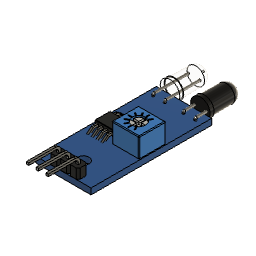
HW-201 v4 (Autodesk Fusion 360 design; units mm, degrees)
Autodesk Fusion 360 part; units mm, degrees
note: some values were not read from the file. Chosen so that the rebuilt part matches the saved one: which bodies a step acts on. Set by a fixed rule: which sketch regions a step uses.
sketch "Sketch1" plane through (0, 0, 0) normal (0, 0, 1) x (1, 0, 0)
  line L0 (7.1, 15.5) -> (-7.1, 15.5)
  line L1 (-7.1, 15.5) -> (-7.1, -15.5)
  line L2 (-7.1, -15.5) -> (7.1, -15.5)
  line L3 (7.1, -15.5) -> (7.1, 15.5)
  line L4 (7.1, 15.5) -> (-7.1, -15.5) construction
  line L5 (-7.1, 15.5) -> (7.1, -15.5) construction
  circle A0 centre (0, -10.4) radius 1.5
  line L6 (0, -10.4) -> (0, -15.5) construction
  dimension "d1" = 14.2
  dimension "d2" = 31
  dimension "d3" = 3
  dimension "d4" = 5.1
  constraint horizontal L0
  constraint perpendicular L0 L1
  constraint parallel L0 L2
  constraint parallel L1 L3
  constraint coincident L4 origin
  constraint coincident L5 origin
  constraint coincident A0.centre L6.start
  constraint midpoint L2 L6.end
  constraint vertical L6
  measures "d1" distance of L1.end L2.end
  measures "d2" distance of L0.end L1.end
  measures "d3" diameter of A0
  measures "d4" distance of A0.centre L6.end
extrude "Extrude1" add sketch "Sketch1" along normal blind 1.54 contours L0 L1 L2 L3 picked at (0.037365, 7.365269) makes body 1
sketch "Sketch2" plane through (0, 0, 1.54) normal (0, 0, 1) x (-1, 0, 0)
  circle A0 centre (0, 10.4) radius 1.5
  line L0 (-7.1, 15.5) -> (-7.1, -15.5)
  line L1 (-7.1, -15.5) -> (7.1, -15.5)
  line L2 (7.1, -15.5) -> (7.1, 15.5)
  line L3 (7.1, 15.5) -> (-7.1, 15.5)
  line L4 (-1.75, 12.95) -> (-3.25, 12.95)
  line L5 (-3.25, 12.95) -> (-3.25, 15.45) construction
  line L6 (-3.25, 15.45) -> (-1.75, 15.45)
  line L7 (-1.75, 15.45) -> (-1.75, 12.95) construction
  line L8 (-1.25, 13.45) -> (-3.75, 13.45) construction
  line L9 (-3.75, 13.45) -> (-3.75, 14.95)
  line L10 (-3.75, 14.95) -> (-1.25, 14.95) construction
  line L11 (-1.25, 14.95) -> (-1.25, 13.45)
  line L12 (1.25, 13.45) -> (-1.25, 13.45) construction
  line L13 (-1.25, 13.45) -> (-1.25, 14.95)
  line L14 (-1.25, 14.95) -> (1.25, 14.95) construction
  line L15 (1.25, 14.95) -> (1.25, 13.45)
  line L16 (0.75, 12.95) -> (-0.75, 12.95)
  line L17 (-0.75, 12.95) -> (-0.75, 15.45) construction
  line L18 (-0.75, 15.45) -> (0.75, 15.45)
  line L19 (0.75, 15.45) -> (0.75, 12.95) construction
  line L20 (3.75, 13.45) -> (1.25, 13.45) construction
  line L21 (1.25, 13.45) -> (1.25, 14.95)
  line L22 (1.25, 14.95) -> (3.75, 14.95) construction
  line L23 (3.75, 14.95) -> (3.75, 13.45)
  line L24 (3.25, 12.95) -> (1.75, 12.95)
  line L25 (1.75, 12.95) -> (1.75, 15.45) construction
  line L26 (1.75, 15.45) -> (3.25, 15.45)
  line L27 (3.25, 15.45) -> (3.25, 12.95) construction
  line L28 (0.75, 12.95) -> (1.25, 13.45)
  line L29 (1.75, 12.95) -> (1.25, 13.45)
  line L30 (3.25, 12.95) -> (3.75, 13.45)
  line L31 (3.75, 14.95) -> (3.25, 15.45)
  line L32 (1.75, 15.45) -> (1.25, 14.95)
  line L33 (1.25, 14.2) -> (3.75, 14.2) construction
  line L34 (2.5, 12.95) -> (2.5, 15.45) construction
  line L35 (0, 12.95) -> (0, 15.45) construction
  line L36 (1.25, 14.2) -> (-1.25, 14.2) construction
  line L37 (-0.75, 12.95) -> (-1.25, 13.45)
  line L38 (-1.25, 14.95) -> (-0.75, 15.45)
  line L39 (1.25, 14.95) -> (0.75, 15.45)
  line L40 (-1.25, 13.45) -> (-1.75, 12.95)
  line L41 (-3.25, 12.95) -> (-3.75, 13.45)
  line L42 (-3.75, 14.95) -> (-3.25, 15.45)
  line L43 (-1.75, 15.45) -> (-1.25, 14.95)
  line L44 (-2.5, 12.95) -> (-2.5, 15.45) construction
  line L45 (-1.25, 14.2) -> (-3.75, 14.2) construction
  line L46 (0, 15.5) -> (0, 14.2) construction
  dimension "d7" = 45
  dimension "d8" = 2.5
  dimension "d9" = 2.5
  dimension "d10" = 2.5
  dimension "d11" = 2.5
  dimension "d12" = 2.5
  dimension "d13" = 2.5
  dimension "d14" = 45
  dimension "d15" = 45
  dimension "d16" = 0.5
  dimension "d17" = 0.5
  dimension "d18" = 0.5
  dimension "d20" = 0.05
  constraint horizontal L4
  constraint vertical L5
  constraint horizontal L6
  constraint vertical L7
  constraint horizontal L8
  constraint vertical L9
  constraint horizontal L10
  constraint vertical L11
  constraint horizontal L12
  constraint vertical L13
  constraint horizontal L14
  constraint vertical L15
  constraint horizontal L16
  constraint vertical L17
  constraint horizontal L18
  constraint vertical L19
  constraint horizontal L20
  constraint vertical L21
  constraint horizontal L22
  constraint vertical L23
  constraint horizontal L24
  constraint vertical L25
  constraint horizontal L26
  constraint vertical L27
  constraint midpoint L21 L33.start
  constraint midpoint L23 L33.end
  constraint midpoint L24 L34.start
  constraint midpoint L26 L34.end
  constraint midpoint L16 L35.start
  constraint perpendicular L16 L35
  constraint midpoint L15 L33.start
  constraint midpoint L13 L36.end
  constraint perpendicular L13 L36
  constraint midpoint L4 L44.start
  constraint midpoint L6 L44.end
  constraint midpoint L11 L36.end
  constraint midpoint L9 L45.end
  constraint midpoint L35 L36
  constraint midpoint L44 L45
  constraint midpoint L33 L34
  constraint coincident L18 L35.end
  constraint collinear L11 L13
  constraint collinear L15 L21
  constraint collinear L4 L16
  constraint collinear L16 L24
  constraint midpoint L3 L46.start
  constraint midpoint L35 L46.end
  constraint vertical L46
  measures "d7" angle of L19 L28
  measures "d8" distance of L8.start L8.end
  measures "d9" distance of L44.start L44.end
  measures "d10" distance of L16.end L17.end
  measures "d11" distance of L12.start L8.start
  measures "d12" distance of L20.start L12.start
  measures "d13" distance of L24.end L25.end
  measures "d14" angle of L7 L40
  measures "d15" angle of L27 L30
  measures "d16" distance of L15 L19
  measures "d17" distance of L7 L11
  measures "d18" distance of L21 L25
  measures "d20" distance of L3 L18
sketch "Sketch3" plane through (0, 0, 1.54) normal (0, 0, 1) x (1, 0, 0)
  line L0 (-0.15, 3.95) -> (6.85, 3.95)
  line L1 (6.85, 3.95) -> (6.85, -2.9)
  line L2 (6.85, -2.9) -> (-0.15, -2.9)
  line L3 (-0.15, -2.9) -> (-0.15, 3.95)
  line L4 (-7.1, -15.5) -> (7.1, -15.5)
  line L5 (7.1, -15.5) -> (7.1, 15.5)
  dimension "d21" = 6.85
  dimension "d22" = 7
  dimension "d23" = 19.45
  dimension "d24" = 0.25
  constraint horizontal L0
  constraint vertical L1
  constraint horizontal L2
  constraint vertical L3
  measures "d21" distance of L0.end L1.end
  measures "d22" distance of L0.start L0.end
  measures "d23" distance of L0 L4
  measures "d24" distance of L1 L5
extrude "Extrude2" add sketch "Sketch3" along normal blind 5 separate body contours L0 L1 L2 L3 picked at (2.183333, 1.666667) makes body 2
sketch "Sketch4" plane through (0, 0, 6.54) normal (0, 0, 1) x (-1, 0, 0)
  line L0 (0.15, 2.9) -> (-6.85, 2.9)
  line L1 (-6.85, 2.9) -> (-6.85, -3.95)
  line L2 (-6.85, -3.95) -> (0.15, -3.95)
  line L3 (0.15, -3.95) -> (0.15, 2.9)
  line L4 (0.15, -0.525) -> (-6.85, -0.525) construction
  line L5 (-3.35, -3.95) -> (-3.35, 2.9) construction
  circle A0 centre (-3.35, -0.525) radius 1.75
  line L6 (-3.25, -3.272141) -> (-3.45, -3.272141)
  line L7 (-3.45, -3.272141) -> (-3.45, -2.272141)
  line L8 (-3.45, -2.272141) -> (-3.25, -2.272141)
  line L9 (-3.25, -2.272141) -> (-3.25, -3.272141)
  line L10 (-3.35, -3.272141) -> (-3.35, -2.272141) construction
  line L11 (-2.063032, -2.954093) -> (-2.563032, -2.088068)
  line L12 (-2.389827, -1.988068) -> (-1.889827, -2.854093)
  line L13 (-1.889827, -2.854093) -> (-2.063032, -2.954093)
  line L14 (-1.020907, -1.985173) -> (-1.886932, -1.485173)
  line L15 (-1.786932, -1.311968) -> (-0.920907, -1.811968)
  line L16 (-0.920907, -1.811968) -> (-1.020907, -1.985173)
  line L17 (-0.602859, -0.625) -> (-1.602859, -0.625)
  line L18 (-1.602859, -0.425) -> (-0.602859, -0.425)
  line L19 (-0.602859, -0.425) -> (-0.602859, -0.625)
  line L20 (-0.920907, 0.761968) -> (-1.786932, 0.261968)
  line L21 (-1.886932, 0.435173) -> (-1.020907, 0.935173)
  line L22 (-1.020907, 0.935173) -> (-0.920907, 0.761968)
  line L23 (-4.810173, -2.854093) -> (-4.310173, -1.988068)
  line L24 (-4.136968, -2.088068) -> (-4.636968, -2.954093)
  line L25 (-4.636968, -2.954093) -> (-4.810173, -2.854093)
  line L26 (-1.889827, 1.804093) -> (-2.389827, 0.938068)
  line L27 (-2.563032, 1.038068) -> (-2.063032, 1.904093)
  line L28 (-2.063032, 1.904093) -> (-1.889827, 1.804093)
  line L29 (-3.25, 2.222141) -> (-3.25, 1.222141)
  line L30 (-3.45, 1.222141) -> (-3.45, 2.222141)
  line L31 (-3.45, 2.222141) -> (-3.25, 2.222141)
  line L32 (-4.636968, 1.904093) -> (-4.136968, 1.038068)
  line L33 (-4.310173, 0.938068) -> (-4.810173, 1.804093)
  line L34 (-4.810173, 1.804093) -> (-4.636968, 1.904093)
  dimension "d27" = 3.5
  dimension "d28" = 0.2
  dimension "d29" = 1
  dimension "d31" = 360
  constraint midpoint L3 L4.start
  constraint midpoint L1 L4.end
  constraint midpoint L2 L5.start
  constraint midpoint L0 L5.end
  constraint midpoint L4 A0.centre
  constraint horizontal L6
  constraint vertical L7
  constraint horizontal L8
  constraint vertical L9
  constraint perpendicular L8 L10
  measures "d27" diameter of A0
extrude "Extrude3" cut sketch "Sketch4" against normal blind 2 contours A0 L8 picked at (-2.629228, -0.607791) bodies 2
extrude "Extrude4" cut sketch "Sketch4" against normal blind 0.1 contours A0 L17 L18 L19 | A0 L20 L21 L22 | A0 L14 L15 L16 | A0 L26 L27 L28 | A0 L11 L12 L13 | A0 L29 L30 L31 | A0 L6 L7 L9 | A0 L32 L33 L34 | A0 L23 L24 L25 picked at (-0.93524, -0.525) picked at (-1.25329, 0.6727) picked at (-1.264406, -1.741954) picked at (-2.1523, 1.57171) picked at (-2.133046, -2.610594) picked at (-3.361116, 1.889654) picked at (-3.338884, -2.939654) picked at (-4.5477, 1.57171) picked at (-4.5477, -2.62171) bodies 2
sketch "Sketch5" plane through (0, 0, 4.54) normal (0, 0, 1) x (-1, 0, 0)
  line L0 (-3.45, -2.272141) -> (-3.25, -2.272141)
  arc A0 (-3.25, -2.272141) -> (-3.45, -2.272141) centre (-3.35, -0.525) ccw
  circle A1 centre (-3.35, -0.525) radius 1.747141
  constraint concentric A0 A1
  constraint tangent L0 A1
extrude "Extrude5" add sketch "Sketch5" along normal blind 1.6 separate body contours L0 A0 A1 picked at (-3.907573, -0.499504) makes body 3
sketch "Sketch6" plane through (0, 0, 6.14) normal (0, 0, 1) x (-1, 0, 0)
  circle A0 centre (-3.35, -0.525) radius 1.747141
  line L0 (-5.097141, -0.8698) -> (-5.097141, -0.1802)
  line L1 (-1.602859, -0.1802) -> (-1.602859, -0.8698)
  line L2 (-3.01881, -2.272141) -> (-3.68119, -2.272141)
  line L3 (-3.68119, 1.222141) -> (-3.01881, 1.222141)
  circle A1 centre (-3.35, -0.525) radius 1.747141
  line L4 (-3.35, -0.525) -> (-3.35, -2.272141) construction
  line L5 (-3.35, -0.525) -> (-1.602859, -0.525) construction
  line L6 (-3.01881, -2.272141) -> (-3.01881, -0.8698)
  line L7 (-3.01881, -0.1802) -> (-3.01881, 1.222141)
  line L8 (-3.68119, 1.222141) -> (-3.68119, -0.1802)
  line L9 (-3.68119, -0.8698) -> (-3.68119, -2.272141)
  line L10 (-1.602859, -0.8698) -> (-3.01881, -0.8698)
  line L11 (-3.68119, -0.8698) -> (-5.097141, -0.8698)
  line L12 (-5.097141, -0.1802) -> (-3.68119, -0.1802)
  line L13 (-3.01881, -0.1802) -> (-1.602859, -0.1802)
  constraint vertical L8
  constraint horizontal L10
  constraint perpendicular L0 L10
  constraint perpendicular L0 L12
  constraint vertical L6
  constraint horizontal L2
  constraint vertical L1
  constraint horizontal L3
  constraint concentric A0 A1
  constraint coincident A0.centre A1.centre
  constraint vertical L4
  constraint horizontal L5
  constraint tangent L2 A1
  constraint tangent L1 A1
  constraint tangent L3 A1
  constraint tangent L0 A1
  constraint collinear L6 L7
  constraint collinear L8 L9
  constraint collinear L10 L11
  constraint collinear L12 L13
extrude "Extrude6" cut sketch "Sketch6" against normal blind 0.5 contours A0 A1 L6 L7 L8 L9 L10 L11 L12 L13 picked at (-2.546827, -0.525) bodies 3
extrude "Extrude7" add sketch "Sketch2" along normal blind 2.5 separate body contours L4 L6 L9 L11 L13 L40 L41 L42 L43 | L11 L13 L15 L16 L18 L21 L28 L37 L38 L39 | L15 L21 L23 L24 L26 L29 L30 L31 L32 picked at (-2.75, 14.616667) picked at (-0.083333, 13.95) picked at (2.75, 13.783333) makes body 4
sketch "Sketch7" plane through (0, 0, 4.04) normal (0, 0, 1) x (-1, 0, 0)
  line L0 (0.75, 12.95) -> (1.25, 13.45)
  line L1 (1.25, 13.45) -> (1.75, 12.95)
  line L2 (1.75, 12.95) -> (3.25, 12.95)
  line L3 (3.25, 12.95) -> (3.75, 13.45)
  line L4 (3.75, 13.45) -> (3.75, 14.95)
  line L5 (3.75, 14.95) -> (3.25, 15.45)
  line L6 (3.25, 15.45) -> (1.75, 15.45)
  line L7 (1.75, 15.45) -> (1.25, 14.95)
  line L8 (1.25, 14.95) -> (0.75, 15.45)
  line L9 (0.75, 15.45) -> (-0.75, 15.45)
  line L10 (-0.75, 15.45) -> (-1.25, 14.95)
  line L11 (-1.25, 14.95) -> (-1.75, 15.45)
  line L12 (-1.75, 15.45) -> (-3.25, 15.45)
  line L13 (-3.25, 15.45) -> (-3.75, 14.95)
  line L14 (-3.75, 14.95) -> (-3.75, 13.45)
  line L15 (-3.75, 13.45) -> (-3.25, 12.95)
  line L16 (-3.25, 12.95) -> (-1.75, 12.95)
  line L17 (-1.75, 12.95) -> (-1.25, 13.45)
  line L18 (-1.25, 13.45) -> (-0.75, 12.95)
  line L19 (-0.75, 12.95) -> (0.75, 12.95)
  line L20 (2.8, 13.9) -> (2.2, 13.9)
  line L21 (2.2, 13.9) -> (2.2, 14.5)
  line L22 (2.2, 14.5) -> (2.8, 14.5)
  line L23 (2.8, 14.5) -> (2.8, 13.9)
  line L24 (0.3, 13.9) -> (-0.3, 13.9)
  line L25 (-0.3, 13.9) -> (-0.3, 14.5)
  line L26 (-0.3, 14.5) -> (0.3, 14.5)
  line L27 (0.3, 14.5) -> (0.3, 13.9)
  line L28 (-2.2, 13.9) -> (-2.8, 13.9)
  line L29 (-2.8, 13.9) -> (-2.8, 14.5)
  line L30 (-2.8, 14.5) -> (-2.2, 14.5)
  line L31 (-2.2, 14.5) -> (-2.2, 13.9)
  line L32 (2.5, 12.95) -> (2.5, 15.45) construction
  line L33 (3.75, 14.2) -> (-3.75, 14.2) construction
  line L34 (-2.5, 12.95) -> (-2.5, 15.45) construction
  line L35 (0, 12.95) -> (0, 15.45) construction
  line L36 (-2.5, 13.9) -> (-2.5, 14.5) construction
  line L37 (0.3, 14.2) -> (-0.3, 14.2) construction
  line L38 (2.5, 14.5) -> (2.5, 13.9) construction
  line L39 (0, 14.5) -> (0, 13.9) construction
  dimension "d42" = 0.6
  constraint horizontal L20
  constraint vertical L21
  constraint horizontal L22
  constraint vertical L23
  constraint horizontal L24
  constraint vertical L25
  constraint horizontal L26
  constraint vertical L27
  constraint horizontal L28
  constraint vertical L29
  constraint horizontal L30
  constraint vertical L31
  constraint equal L28 L29
  constraint equal L24 L25
  constraint equal L20 L21
  constraint equal L20 L24
  constraint equal L24 L28
  constraint midpoint L2 L32.start
  constraint midpoint L6 L32.end
  constraint midpoint L4 L33.start
  constraint midpoint L14 L33.end
  constraint midpoint L16 L34.start
  constraint midpoint L12 L34.end
  constraint midpoint L19 L35.start
  constraint midpoint L9 L35.end
  constraint midpoint L28 L36.start
  constraint midpoint L30 L36.end
  constraint perpendicular L30 L36
  constraint midpoint L27 L37.start
  constraint midpoint L25 L37.end
  constraint midpoint L22 L38.start
  constraint midpoint L20 L38.end
  constraint perpendicular L20 L38
  constraint collinear L24 L28
  constraint collinear L20 L24
  constraint collinear L34 L36
  constraint midpoint L26 L39.start
  constraint midpoint L24 L39.end
  constraint collinear L35 L39
  constraint collinear L32 L38
  constraint collinear L33 L37
  measures "d42" distance of L28.start L28.end
sketch "Sketch8" plane through (3.75, 0, 0) normal (1, 0, 0) x (0, 1, 0)
  line L0 (-14.95, 1.54) -> (-13.45, 1.54)
  line L1 (-13.45, 1.54) -> (-13.45, 4.04)
  line L2 (-13.45, 4.04) -> (-14.95, 4.04)
  line L3 (-14.95, 4.04) -> (-14.95, 1.54)
  line L4 (-14.2, 4.04) -> (-14.2, 4.54)
  line L5 (-15.2, 5.54) -> (-22.2, 5.54)
  arc A0 (-14.2, 4.54) -> (-15.2, 5.54) centre (-15.2, 4.54) ccw
  point P0 (-14.2, 5.54)
  dimension "d43" = 1.5
  dimension "d44" = 8
  dimension "d45" = 1
  constraint midpoint L2 L4.start
  constraint perpendicular L2 L4
  constraint perpendicular L4 L5
  constraint coincident P0 L5
  constraint coincident P0 L4
  constraint tangent L5 A0
  constraint tangent L4 A0
  measures "d43" distance of L4.start P0
  measures "d44" distance of P0 L5.end
  measures "d45" radius of A0
sweep "Sweep1" add profiles "Sketch7" path "Sketch8" along L4 A0 L5 section 1 contours L20 L21 L22 L23 | L24 L25 L26 L27 | L28 L29 L30 L31 picked at (2.6, 14.1) picked at (0.1, 14.1) picked at (-2.4, 14.1) separate body makes body 5 at (2.8, -17.533333, 5.44) makes body 6 at (0.3, -17.533333, 5.44) makes body 7 at (-2.2, -17.533333, 5.44)
sketch "Sketch9" plane through (7.1, 0, 0) normal (1, 0, 0) x (0, 1, 0)
  line L0 (-15.5, 0) -> (15.5, 0)
  line L1 (15.5, 0) -> (15.5, 1.54)
  line L2 (15.5, 1.54) -> (-15.5, 1.54)
  line L3 (-15.5, 1.54) -> (-15.5, 0)
  line L4 (13, -2.3) -> (13, 2.04) construction
  line L5 (13.2, 2.04) -> (22, 2.04)
  line L6 (13, 1.84) -> (13, 1.54)
  line L7 (13, 0) -> (13, -2.3)
  arc A0 (13.2, 2.04) -> (13, 1.84) centre (13.2, 1.84) ccw
  dimension "d52" = 2.5
  dimension "d53" = 0.5
  dimension "d54" = 2.3
  dimension "d55" = 9
  dimension "d69" = 0.2
  constraint perpendicular L0 L4
  constraint perpendicular L4 L5
  constraint coincident L4 L6.end
  constraint coincident L2 L6.end
  constraint coincident L0 L7.start
  constraint coincident L4 L7.start
  constraint coincident L4.end L6
  constraint coincident L4.end L5
  constraint tangent L5 A0
  measures "d52" distance of L1 L4
  measures "d53" distance of L2 L5
  measures "d54" distance of L0 L4.start
  measures "d55" distance of L4.end L5.end
  measures "d69" radius of A0
sketch "Sketch10" plane through (0, 0, 1.54) normal (0, 0, 1) x (-1, 0, 0)
  circle A0 centre (0, 10.4) radius 1.5
  line L0 (-7.1, 15.5) -> (-7.1, -15.5)
  line L1 (-7.1, -15.5) -> (7.1, -15.5)
  line L2 (7.1, -15.5) -> (7.1, 15.5)
  line L3 (7.1, 15.5) -> (-7.1, 15.5)
  line L4 (-3.9, -14.5) -> (-6.9, -14.5)
  line L5 (-6.9, -14.5) -> (-6.9, -11.5)
  line L6 (-6.9, -11.5) -> (-3.9, -11.5)
  line L7 (-3.9, -11.5) -> (-3.9, -14.5)
  line L8 (-0.9, -14.5) -> (-3.9, -14.5)
  line L9 (-3.9, -14.5) -> (-3.9, -11.5)
  line L10 (-3.9, -11.5) -> (-0.9, -11.5)
  line L11 (-0.9, -11.5) -> (-0.9, -14.5)
  line L12 (3.9, -14.5) -> (0.9, -14.5)
  line L13 (0.9, -14.5) -> (0.9, -11.5)
  line L14 (0.9, -11.5) -> (3.9, -11.5)
  line L15 (3.9, -11.5) -> (3.9, -14.5)
  line L16 (6.9, -14.5) -> (3.9, -14.5)
  line L17 (3.9, -14.5) -> (3.9, -11.5)
  line L18 (3.9, -11.5) -> (6.9, -11.5)
  line L19 (6.9, -11.5) -> (6.9, -14.5)
  line L20 (-7.1, -13) -> (7.1, -13) construction
  line L21 (-7.1, -13.2) -> (-7.1, -22)
  line L22 (-5.1, -13.3) -> (-5.7, -13.3) construction
  line L23 (-5.7, -13.3) -> (-5.7, -12.7) construction
  line L24 (-5.7, -12.7) -> (-5.1, -12.7) construction
  line L25 (-5.1, -12.7) -> (-5.1, -13.3) construction
  line L26 (-2.1, -13.3) -> (-2.7, -13.3) construction
  line L27 (-2.7, -13.3) -> (-2.7, -12.7) construction
  line L28 (-2.7, -12.7) -> (-2.1, -12.7) construction
  line L29 (-2.1, -12.7) -> (-2.1, -13.3) construction
  line L30 (2.7, -13.3) -> (2.1, -13.3) construction
  line L31 (2.1, -13.3) -> (2.1, -12.7) construction
  line L32 (2.1, -12.7) -> (2.7, -12.7) construction
  line L33 (2.7, -12.7) -> (2.7, -13.3) construction
  line L34 (5.7, -13.3) -> (5.1, -13.3) construction
  line L35 (5.1, -13.3) -> (5.1, -12.7) construction
  line L36 (5.1, -12.7) -> (5.7, -12.7) construction
  line L37 (5.7, -12.7) -> (5.7, -13.3) construction
  line L38 (-2.4, -14.5) -> (-2.4, -11.5) construction
  line L39 (-5.4, -14.5) -> (-5.4, -11.5) construction
  line L40 (2.4, -14.5) -> (2.4, -11.5) construction
  line L41 (5.4, -14.5) -> (5.4, -11.5) construction
  line L42 (5.7, -13) -> (5.1, -13) construction
  line L43 (5.4, -13.3) -> (5.4, -12.7) construction
  line L44 (2.4, -13.3) -> (2.4, -12.7) construction
  line L45 (2.7, -13) -> (2.1, -13) construction
  line L46 (-2.4, -13.3) -> (-2.4, -12.7) construction
  line L47 (-5.4, -13.3) -> (-5.4, -12.7) construction
  circle A1 centre (5.4, -13) radius 0.3
  circle A2 centre (2.4, -13) radius 0.3
  circle A3 centre (-2.4, -13) radius 0.3
  circle A4 centre (-5.4, -13) radius 0.3
  line L48 (4, -11.6) -> (6.8, -11.6)
  line L49 (6.8, -11.6) -> (6.8, -14.4)
  line L50 (6.8, -14.4) -> (4, -14.4)
  line L51 (4, -14.4) -> (4, -11.6)
  line L52 (1, -11.6) -> (3.8, -11.6)
  line L53 (3.8, -11.6) -> (3.8, -14.4)
  line L54 (3.8, -14.4) -> (1, -14.4)
  line L55 (1, -14.4) -> (1, -11.6)
  line L56 (-3.8, -11.6) -> (-1, -11.6)
  line L57 (-1, -11.6) -> (-1, -14.4)
  line L58 (-1, -14.4) -> (-3.8, -14.4)
  line L59 (-3.8, -14.4) -> (-3.8, -11.6)
  line L60 (-6.8, -11.6) -> (-4, -11.6)
  line L61 (-4, -11.6) -> (-4, -14.4)
  line L62 (-4, -14.4) -> (-6.8, -14.4)
  line L63 (-6.8, -14.4) -> (-6.8, -11.6)
  point P0 (-7.1, -13)
  dimension "d56" = 3
  dimension "d57" = 3
  dimension "d58" = 3
  dimension "d59" = 1
  dimension "d60" = 0.2
  dimension "d61" = 3
  dimension "d62" = 3
  dimension "d63" = 0.2
  dimension "d64" = 0.6
  dimension "d65" = 0.1
  dimension "d66" = 0.1
  dimension "d67" = 0.1
  dimension "d68" = 0.1
  constraint horizontal L4
  constraint vertical L5
  constraint horizontal L6
  constraint vertical L7
  constraint horizontal L8
  constraint vertical L9
  constraint horizontal L10
  constraint vertical L11
  constraint horizontal L12
  constraint vertical L13
  constraint horizontal L14
  constraint vertical L15
  constraint horizontal L16
  constraint vertical L17
  constraint horizontal L18
  constraint vertical L19
  constraint collinear L15 L17
  constraint collinear L14 L18
  constraint collinear L12 L16
  constraint perpendicular L2 L20
  constraint collinear L8 L12
  constraint collinear L4 L12
  constraint collinear L10 L14
  constraint collinear L6 L10
  constraint collinear L7 L9
  constraint horizontal L22
  constraint vertical L23
  constraint horizontal L24
  constraint vertical L25
  constraint horizontal L26
  constraint vertical L27
  constraint horizontal L28
  constraint vertical L29
  constraint horizontal L30
  constraint vertical L31
  constraint horizontal L32
  constraint vertical L33
  constraint horizontal L34
  constraint vertical L35
  constraint horizontal L36
  constraint vertical L37
  constraint equal L34 L35
  constraint equal L30 L34
  constraint equal L30 L31
  constraint equal L26 L30
  constraint equal L26 L27
  constraint equal L25 L27
  constraint equal L22 L25
  constraint collinear L30 L34
  constraint collinear L26 L30
  constraint collinear L22 L26
  constraint midpoint L8 L38.start
  constraint midpoint L10 L38.end
  constraint midpoint L4 L39.start
  constraint midpoint L6 L39.end
  constraint midpoint L12 L40.start
  constraint midpoint L14 L40.end
  constraint midpoint L16 L41.start
  constraint midpoint L18 L41.end
  constraint midpoint L37 L42.start
  constraint midpoint L35 L42.end
  constraint midpoint L34 L43.start
  constraint midpoint L36 L43.end
  constraint perpendicular L36 L43
  constraint midpoint L30 L44.start
  constraint midpoint L32 L44.end
  constraint midpoint L33 L45.start
  constraint midpoint L31 L45.end
  constraint collinear L20 L42
  constraint midpoint L26 L46.start
  constraint midpoint L28 L46.end
  constraint collinear L38 L46
  constraint midpoint L22 L47.start
  constraint midpoint L24 L47.end
  constraint perpendicular L24 L47
  constraint collinear L39 L47
  constraint collinear L40 L44
  constraint collinear L41 L43
  constraint midpoint L42 A1.centre
  constraint coincident L43.start A1
  constraint midpoint L40 A2.centre
  constraint coincident L44.start A2
  constraint midpoint L38 A3.centre
  constraint coincident L46.start A3
  constraint midpoint L47 A4.centre
  constraint coincident L47.start A4
  constraint coincident L2 L20.end
  constraint coincident P0 L20.start
  measures "d56" distance of L16.start L12.start
  measures "d57" distance of L12.start L12.end
  measures "d58" distance of L16.start L18.end
  measures "d59" distance of L1 L16
  measures "d60" distance of L2 L19
  measures "d61" distance of L4.start L4.end
  measures "d62" distance of L8.start L4.start
  measures "d63" distance of L5 L21
  measures "d64" distance of L32.end L31
sweep "Sweep2" add profiles "Sketch10" path "Sketch9" along L5 A0 L6 section 1 contours A1 | A2 | A3 | A4 picked at (5.272872, -13.056332) picked at (2.488251, -12.931983) picked at (-2.311749, -12.931983) picked at (-5.527128, -13.056332) separate body makes body 8 at (5.630983, 19.066667, 1.848567) makes body 9 at (2.630983, 19.066667, 1.848567) makes body 10 at (-5.169017, 19.066667, 1.848567) makes body 11 at (-2.169017, 19.066667, 1.848567)
ref_plane "WorkPlane1" through (0, 15.8, 0.77) normal (0, 1, 0) x (-1, 0, 0)
sketch "Sketch11" plane through (0, 15.8, 0.77) normal (0, 1, 0) x (1, 0, 0)
  circle A0 centre (5.4, -1.27) radius 0.3
  circle A1 centre (2.4, -1.27) radius 0.3
  line L0 (7.1, 0.77) -> (-7.1, 0.77)
  line L1 (-7.1, 0.77) -> (-7.1, -0.77)
  line L2 (-7.1, -0.77) -> (7.1, -0.77)
  line L3 (7.1, -0.77) -> (7.1, 0.77)
  line L4 (5.4, -1.27) -> (2.4, -1.27) construction
  line L5 (3.9, -3.77) -> (3.9, 1.23) construction
  circle A2 centre (3.9, -1.27) radius 2.5
  circle A3 centre (-2.4, -1.27) radius 0.3
  circle A4 centre (-5.4, -1.27) radius 0.3
  line L6 (-7.1, 0.77) -> (7.1, 0.77)
  line L7 (7.1, 0.77) -> (7.1, -0.77)
  line L8 (7.1, -0.77) -> (-7.1, -0.77)
  line L9 (-7.1, -0.77) -> (-7.1, 0.77)
  line L10 (-2.4, -1.27) -> (-5.4, -1.27) construction
  line L11 (-3.9, -3.77) -> (-3.9, 1.23) construction
  circle A5 centre (-3.9, -1.27) radius 2.5
  dimension "d77" = 5
  dimension "d78" = 5
  constraint coincident A0.centre L4.start
  constraint coincident A1.centre L4.end
  constraint perpendicular L2 L5
  constraint midpoint L4 L5
  constraint midpoint L4 A2.centre
  constraint coincident L5.start A2
  constraint coincident A3.centre L10.start
  constraint coincident A4.centre L10.end
  constraint perpendicular L0 L11
  constraint midpoint L10 L11
  constraint midpoint L10 A5.centre
  constraint coincident L11.start A5
  measures "d77" distance of L5.start L5.end
  measures "d78" distance of L11.start L11.end
extrude "Extrude8" add sketch "Sketch11" along normal blind 1 separate body contours A0 | A1 | L0 L2 A2 L6 L8 | L0 A2 L6 | L2 A2 L8 | L0 L2 L6 L8 A5 | L0 L6 A5 | L2 L8 A5 | A3 | A4 picked at (5.35, -1.161617) picked at (2.407473, -1.17028) picked at (4.490335, -0.221416) picked at (3.729996, 1.024614) picked at (3.876665, -2.215671) picked at (-3.309665, -0.221416) picked at (-3.515646, 0.829403) picked at (-3.923335, -2.215671) picked at (-2.407473, -1.17028) picked at (-5.45, -1.161617) makes body 12 at (-4.456597, 15.8, 2.937156) makes body 13 at (4.559506, 16.8, 2.896767)
sketch "Sketch12" plane through (0, 16.8, 0) normal (0, 1, 0) x (-1, 0, 0)
  circle A0 centre (-3.9, 2.04) radius 2.5
  circle A1 centre (-3.9, 2.04) radius 2.3
  dimension "d81" = -0.2
extrude "Extrude9" add sketch "Sketch12" along normal blind 7.6 draft -0.6 separate body contours A1 picked at (-3.679192, 2.561466) makes body 14
fillet "Fillet1" radius 2 1 edges at (5.970149, 24.4, 2.842935) on bodies 14
combine "Combine1" operation add target body 14 tool bodies 13
sketch "Sketch14" plane through (0, 16.8, 0) normal (0, 1, 0) x (-1, 0, 0)
  circle A0 centre (3.9, 2.04) radius 2.5
  circle A1 centre (3.9, 2.04) radius 2.3
  dimension "d86" = -0.2
extrude "Extrude10" add sketch "Sketch14" along normal blind 7.6 draft -0.6 separate body contours A1 picked at (3.619905, 2.75367) makes body 15
fillet "Fillet2" radius 2 1 faces at (-4.346032, 24.4, 1.305555) on bodies 15
combine "Combine2" operation add target body 12 tool bodies 15
ref_plane "WorkPlane2" through (-6.1, 0, 0.77) normal (-1, 0, 0) x (0, -1, 0)
sketch "Sketch15" plane through (-6.1, 0, 0.77) normal (-1, 0, 0) x (0, 1, 0)
  line L0 (2.6, -2.27) -> (-1.3, -2.27)
  line L1 (-1.3, -2.27) -> (-1.3, -0.77)
  line L2 (-1.3, -0.77) -> (2.6, -0.77)
  line L3 (2.6, -0.77) -> (2.6, -2.27)
  line L4 (3.95, -0.77) -> (-2.9, -0.77)
  line L5 (-2.9, -0.77) -> (-2.9, -5.77)
  line L6 (-2.9, -5.77) -> (3.95, -5.77)
  line L7 (3.95, -5.77) -> (3.95, -0.77)
  line L8 (15.5, -0.77) -> (-15.5, -0.77)
  dimension "d92" = 3.9
  dimension "d93" = 1.5
  dimension "d94" = 1.6
  constraint horizontal L0
  constraint vertical L1
  constraint horizontal L2
  constraint vertical L3
  constraint collinear L2 L8
  measures "d92" distance of L0.start L0.end
  measures "d93" distance of L0.end L1.end
  measures "d94" distance of L1 L5
extrude "Extrude11" add sketch "Sketch15" against normal blind 5 separate body contours L0 L1 L2 L3 L4 L8 picked at (0, -1.77) makes body 16
fillet "Fillet3" radius 0.1 4 edges at (-3.6, -1.3, 1.54) (-3.6, -1.3, 3.04) (-3.6, 2.6, 3.04) (-3.6, 2.6, 1.54) 2 faces at (-6.1, 0, 2.54) (-1.1, 0, 2.54) on bodies 16
sketch "Sketch16" plane through (-6.1, 0, 0) normal (-1, 0, 0) x (0, -1, 0)
  line L0 (-2.5, 1.64) -> (1.2, 1.64)
  line L1 (1.2, 1.64) -> (1.2, 2.94)
  line L2 (1.2, 2.94) -> (-2.5, 2.94)
  line L3 (-2.5, 2.94) -> (-2.5, 1.64)
  line L4 (-2.6, 2.29) -> (-3.5, 2.29)
  line L5 (-2.6, 2.94) -> (-2.6, 1.64)
  line L6 (-3.68, 2.23) -> (-4.6, 1.54)
  line L7 (-15.5, 0) -> (15.5, 0)
  line L8 (15.5, 0) -> (15.5, 1.54)
  line L9 (15.5, 1.54) -> (-15.5, 1.54)
  line L10 (-15.5, 1.54) -> (-15.5, 0)
  arc A0 (-3.5, 2.29) -> (-3.68, 2.23) centre (-3.5, 1.99) ccw
  line L11 (-4.6, 1.54) -> (-5.1, 1.165)
  line L12 (-5.1, 1.165) -> (-5.1, 2.126257) construction
  point P0 (-3.6, 2.29)
  dimension "d100" = 1
  dimension "d101" = 2
  dimension "d102" = 0.3
  dimension "d114" = 0.5
  constraint perpendicular L3 L4
  constraint midpoint L4.start L5
  constraint coincident L6.end L9
  constraint coincident P0 L4
  constraint coincident P0 L6
  constraint tangent L4 A0
  constraint tangent L6 A0
  constraint parallel L6 L11
  constraint vertical L12
  measures "d100" distance of L4.start P0
  measures "d101" horizontal distance of L4.start L6.end
  measures "d102" radius of A0
  measures "d114" distance of L6.end L12
sketch "Sketch17" plane through (0, 2.6, 0) normal (0, 1, 0) x (-1, 0, 0)
  line L0 (6, 1.64) -> (6, 2.94)
  line L1 (6, 2.94) -> (1.2, 2.94)
  line L2 (1.2, 2.94) -> (1.2, 1.64)
  line L3 (1.2, 1.64) -> (6, 1.64)
  line L4 (5.2, 2.54) -> (5.7, 2.54)
  line L5 (5.7, 2.54) -> (5.7, 2.04)
  line L6 (5.7, 2.04) -> (5.2, 2.04)
  line L7 (5.2, 2.04) -> (5.2, 2.54)
  line L8 (6.1, 2.94) -> (6.1, 1.64)
  line L9 (5.7, 2.29) -> (6.1, 2.29) construction
  line L10 (1.5, 2.54) -> (2, 2.54)
  line L11 (2, 2.54) -> (2, 2.04)
  line L12 (2, 2.04) -> (1.5, 2.04)
  line L13 (1.5, 2.04) -> (1.5, 2.54)
  line L14 (2.733333, 2.54) -> (3.233333, 2.54)
  line L15 (3.233333, 2.54) -> (3.233333, 2.04)
  line L16 (3.233333, 2.04) -> (2.733333, 2.04)
  line L17 (2.733333, 2.04) -> (2.733333, 2.54)
  line L18 (3.966667, 2.54) -> (4.466667, 2.54)
  line L19 (4.466667, 2.54) -> (4.466667, 2.04)
  line L20 (4.466667, 2.04) -> (3.966667, 2.04)
  line L21 (3.966667, 2.04) -> (3.966667, 2.54)
  line L22 (1.1, 2.94) -> (1.1, 1.64)
  line L23 (2, 2.29) -> (2.733333, 2.29) construction
  line L24 (3.233333, 2.29) -> (3.966667, 2.29) construction
  line L25 (4.466667, 2.29) -> (5.2, 2.29) construction
  dimension "d103" = 0.5
  dimension "d104" = 0.4
  dimension "d105" = 0.5
  dimension "d107" = 0.4
  constraint horizontal L4
  constraint vertical L5
  constraint horizontal L6
  constraint vertical L7
  constraint midpoint L5 L9.start
  constraint midpoint L8 L9.end
  constraint horizontal L9
  constraint horizontal L10
  constraint vertical L11
  constraint horizontal L12
  constraint vertical L13
  constraint horizontal L14
  constraint vertical L15
  constraint horizontal L16
  constraint vertical L17
  constraint horizontal L18
  constraint vertical L19
  constraint horizontal L20
  constraint vertical L21
  constraint equal L14 L18
  constraint equal L4 L18
  constraint equal L7 L19
  constraint equal L7 L15
  constraint equal L7 L11
  constraint equal L10 L14
  constraint collinear L4 L18
  constraint collinear L14 L18
  constraint collinear L10 L14
  constraint midpoint L11 L23.start
  constraint midpoint L7 L25.end
  constraint equal L24 L25
  constraint equal L23 L24
  measures "d103" distance of L4.start L4.end
  measures "d104" distance of L5 L8
  measures "d105" distance of L4 L6
  measures "d107" distance of L13 L22
sweep "Sweep3" add profiles "Sketch17" path "Sketch16" along L4 A0 L6 L11 section 1 contours L4 L5 L6 L7 | L10 L11 L12 L13 | L14 L15 L16 L17 | L18 L19 L20 L21 picked at (5.533333, 2.373333) picked at (1.833333, 2.206667) picked at (2.9, 2.206667) picked at (4.133333, 2.373333) separate body makes body 17 at (-4.466667, 4.103333, 1.808333) makes body 18 at (-3.233333, 4.103333, 1.808333) makes body 19 at (-5.7, 4.103333, 1.808333) makes body 20 at (-2, 4.103333, 1.808333)
ref_plane "WorkPlane3" through (-3.6, 0.65, 2.29) normal (0, 1, 0) x (0, 0, 1)
mirror "Mirror1" about plane through (-3.6, 0.65, 2.29) normal (0, 1, 0) of "Sweep3" makes body 21 at (-4.466667, -2.803333, 1.808333) makes body 22 at (-3.233333, -2.803333, 1.808333) makes body 23 at (-5.7, -2.803333, 1.808333) makes body 24 at (-2, -2.803333, 1.808333)
fillet "Fillet4" radius 0.2 8 edges at (-0.15, -2.9, 4.04) (-0.15, 3.95, 4.04) (6.85, -2.9, 4.04) (6.85, 3.95, 4.04) (6.85, 0.525, 6.54) (3.35, -2.9, 6.54) (-0.15, 0.525, 6.54) (3.35, 3.95, 6.54) on bodies 2
equation "d9 = d8"
equation "d10 = d9"
equation "d11 = d8"
equation "d12 = d8"
equation "d13 = d9"
equation "d53 = 0.2 mm + 0.3 mm"
equation "d58 = d56"
equation "d61 = d57"
equation "d62 = d61"
equation "d78 = d77"
equation "d105 = d103"
equation "d107 = d104"
named bodies: "PCB", "Pot", "Pot Wheel", "Headers", "VCC Pin", "GND Pin", "Out Pin", "Pin Right", "Pin Left (1)", "Pin Left", "Pin Right (1)", "Glass LED", "Black LED", "Chip", "Leg", "Leg (1)", "Leg (2)", "Leg (3)", "Leg (7)", "Leg (4)", "Leg (5)", "Leg (6)"
